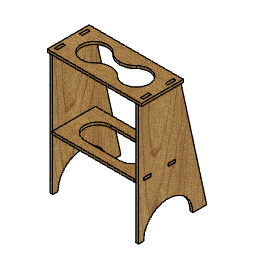
Prototipo_POMPE_2_0 (Autodesk Fusion 360 archive; units mm, degrees)
design "soporte_caños_corte_ v3"
Autodesk Fusion 360 part; units mm, degrees
sketch "Boceto1" plane through (0, 0, 0) normal (0, 0, 1) x (1, 0, 0)
  line L0 (0, 80) -> (0, -80) construction
  line L1 (180, 0) -> (180, -80)
  line L2 (180, 0) -> (180, 80)
  arc A0 (44.5386, -35.4614) -> (-44.5386, -35.4614) centre (0, -80) ccw
  arc A1 (-44.5386, 35.4614) -> (-44.5386, -35.4614) centre (-80, 0) ccw
  arc A2 (-44.5386, 35.4614) -> (44.5386, 35.4614) centre (0, 80) ccw
  arc A3 (44.5386, -35.4614) -> (44.5386, 35.4614) centre (80, 0) ccw
  line L3 (0, 0) -> (84.5309, 0)
  line L4 (-158.4928, 60.1913) -> (-158.4928, 34.434)
  line L5 (-180, 0) -> (-180, -80)
  line L6 (-166.3715, 62.3127) -> (-160.6141, 62.3127)
  line L7 (-180, 0) -> (-180, 80)
  line L8 (-168.4928, 34.434) -> (-168.4928, 60.1913)
  line L9 (-160.6141, 32.3127) -> (-166.3715, 32.3127)
  line L10 (-180, 80) -> (180, 80)
  line L11 (-180, -80) -> (180, -80)
  line L12 (-163.4928, 62.3127) -> (-163.4928, 32.3127)
  line L13 (-166.3715, 62.3127) -> (-160.1055, 62.3127) construction
  arc A4 (-166.3715, 62.3127) -> (-168.4928, 60.1913) centre (-167.4321, 61.252) ccw
  arc A5 (-158.4928, 60.1913) -> (-160.6141, 62.3127) centre (-159.5534, 61.252) ccw
  line L14 (-163.4928, 47.3127) -> (-158.4928, 47.3127)
  arc A6 (-160.6141, 32.3127) -> (-158.4928, 34.434) centre (-159.5534, 33.3733) ccw
  arc A7 (-168.4928, 34.434) -> (-166.3715, 32.3127) centre (-167.4321, 33.3733) ccw
  arc A8 (158.4928, 34.434) -> (160.6141, 32.3127) centre (159.5534, 33.3733) ccw
  line L15 (160.6141, 32.3127) -> (166.3715, 32.3127)
  arc A9 (166.3715, 32.3127) -> (168.4928, 34.434) centre (167.4321, 33.3733) ccw
  line L16 (168.4928, 34.434) -> (168.4928, 60.1913)
  arc A10 (168.4928, 60.1913) -> (166.3715, 62.3127) centre (167.4321, 61.252) ccw
  line L17 (166.3715, 62.3127) -> (160.6141, 62.3127)
  arc A11 (160.6141, 62.3127) -> (158.4928, 60.1913) centre (159.5534, 61.252) ccw
  line L18 (158.4928, 60.1913) -> (158.4928, 34.434)
  line L19 (166.3715, -62.3127) -> (160.6141, -62.3127)
  arc A12 (158.4928, -60.1913) -> (160.6141, -62.3127) centre (159.5534, -61.252) ccw
  line L20 (158.4928, -60.1913) -> (158.4928, -34.434)
  arc A13 (160.6141, -32.3127) -> (158.4928, -34.434) centre (159.5534, -33.3733) ccw
  line L21 (160.6141, -32.3127) -> (166.3715, -32.3127)
  arc A14 (168.4928, -34.434) -> (166.3715, -32.3127) centre (167.4321, -33.3733) ccw
  line L22 (168.4928, -34.434) -> (168.4928, -60.1913)
  arc A15 (166.3715, -62.3127) -> (168.4928, -60.1913) centre (167.4321, -61.252) ccw
  arc A16 (-158.4928, -34.434) -> (-160.6141, -32.3127) centre (-159.5534, -33.3733) ccw
  line L23 (-160.6141, -32.3127) -> (-166.3715, -32.3127)
  arc A17 (-166.3715, -32.3127) -> (-168.4928, -34.434) centre (-167.4321, -33.3733) ccw
  line L24 (-168.4928, -34.434) -> (-168.4928, -60.1913)
  arc A18 (-168.4928, -60.1913) -> (-166.3715, -62.3127) centre (-167.4321, -61.252) ccw
  line L25 (-166.3715, -62.3127) -> (-160.6141, -62.3127)
  arc A19 (-160.6141, -62.3127) -> (-158.4928, -60.1913) centre (-159.5534, -61.252) ccw
  line L26 (-158.4928, -60.1913) -> (-158.4928, -34.434)
  point P0 (-180.15, 0)
  dimension "d29" = 3
  dimension "d37" = 10
  constraint vertical L0
  constraint coincident L3.start origin
  constraint perpendicular L0 L3
  constraint symmetric L0 L1.start L5.start
  constraint symmetric L0 L1.end L5.end
  constraint symmetric L0 L2.end L7.end
  constraint perpendicular L2 L10
  constraint perpendicular L1 L11
  constraint perpendicular L9 L12
  constraint horizontal L13
  constraint symmetric L12 L8.end L4.start
  constraint symmetric L12 L6.start L6.end
  constraint symmetric L12 A4 A5
  constraint midpoint L12 L14.start
  constraint perpendicular L12 L14
  constraint symmetric L8.end L14 L8.start
  constraint symmetric L6.start L14 L9.end
  constraint symmetric A4 L14 A7
  constraint symmetric L6.end L14 L9.start
  constraint symmetric L4.start L14 L4.end
  constraint symmetric A5 L14 A6
  constraint coincident L6 L12.start
  constraint coincident L9 L12.end
  constraint symmetric L0 L8.end L16.end
  constraint symmetric L0 L6.start A10.end
  constraint symmetric L0 A4 A10
  constraint symmetric L0 L6.end L17.end
  constraint symmetric L0 L4.start A11.end
  constraint symmetric L0 A5 A11
  constraint symmetric L0 L4.end A8.start
  constraint symmetric L0 L9.start A8.end
  constraint symmetric L0 A6 A8
  constraint symmetric L0 L9.end L15.end
  constraint symmetric L0 L8.start A9.end
  constraint symmetric L0 A7 A9
  constraint symmetric L3 L8.end L24.end
  constraint symmetric L3 L6.start A18.end
  constraint symmetric L3 A4 A18
  constraint symmetric L3 L6.end L25.end
  constraint symmetric L3 L4.start A19.end
  constraint symmetric L3 A5 A19
  constraint symmetric L3 L4.end A16.start
  constraint symmetric L3 L9.start A16.end
  constraint symmetric L3 A6 A16
  constraint symmetric L3 L9.end L23.end
  constraint symmetric L3 L8.start A17.end
  constraint symmetric L3 A7 A17
  constraint symmetric L3 A8.end A13.start
  constraint symmetric L3 A8.start L20.end
  constraint symmetric L3 A8 A13
  constraint symmetric L3 L15.end L21.end
  constraint symmetric L3 A9.end A14.start
  constraint symmetric L3 A9 A14
  constraint symmetric L3 L16.end L22.end
  constraint symmetric L3 A10.end L19.start
  constraint symmetric L3 A10 A15
  constraint symmetric L3 L17.end L19.end
  constraint symmetric L3 A11.end A12.start
  constraint symmetric L3 A11 A12
  constraint coincident L0.end A0.centre
  constraint coincident L0.start A2.centre
  constraint horizontal L14
  constraint midpoint L4 L14.end
  measures "d29" diameter of A4
  measures "d37" distance of L4 L8
sketch "Boceto2" plane through (0, 0, 0) normal (0, 0, 1) x (1, 0, 0)
  line L0 (-158.6799, -83.0083) -> (0, -83.0083)
  arc A0 (-66.8983, 50.15) -> (-66.8983, -50.15) centre (-66.8983, 0) ccw
  line L1 (-66.8983, 50.15) -> (0, 50.15)
  line L2 (-66.8983, -50.15) -> (0, -50.15)
  line L3 (-158.6799, -62.4727) -> (-158.6799, -83.0083)
  line L4 (-169.0788, -33.0938) -> (-169.0788, -60.3514)
  line L5 (-160.8013, -33.0938) -> (-169.0788, -33.0938)
  line L6 (-169.0788, -60.3514) -> (-160.8013, -60.3514)
  line L7 (0, 0) -> (-158.6799, 0)
  line L8 (0, 0) -> (0, -83.0083)
  line L9 (-158.6799, -30.9725) -> (-158.6799, 0)
  arc A1 (-160.8013, -33.0938) -> (-158.6799, -30.9725) centre (-159.7406, -32.0332) ccw
  line L10 (-158.6799, -33.0938) -> (-159.7406, -32.0332) construction
  line L11 (-169.0788, -46.7226) -> (-158.6799, -46.7226)
  arc A2 (-158.6799, -62.4727) -> (-160.8013, -60.3514) centre (-159.7406, -61.412) ccw
  line L12 (-158.6799, 83.0083) -> (0, 83.0083)
  line L13 (-158.6799, 62.4727) -> (-158.6799, 83.0083)
  arc A3 (-160.8013, 60.3514) -> (-158.6799, 62.4727) centre (-159.7406, 61.412) ccw
  line L14 (-169.0788, 60.3514) -> (-160.8013, 60.3514)
  line L15 (-169.0788, 33.0938) -> (-169.0788, 60.3514)
  line L16 (-160.8013, 33.0938) -> (-169.0788, 33.0938)
  arc A4 (-158.6799, 30.9725) -> (-160.8013, 33.0938) centre (-159.7406, 32.0332) ccw
  line L17 (-158.6799, 30.9725) -> (-158.6799, 0)
  line L18 (158.6799, 83.0083) -> (0, 83.0083)
  line L19 (158.6799, 62.4727) -> (158.6799, 83.0083)
  arc A5 (158.6799, 62.4727) -> (160.8013, 60.3514) centre (159.7406, 61.412) ccw
  line L20 (169.0788, 60.3514) -> (160.8013, 60.3514)
  line L21 (169.0788, 33.0938) -> (169.0788, 60.3514)
  line L22 (160.8013, 33.0938) -> (169.0788, 33.0938)
  arc A6 (160.8013, 33.0938) -> (158.6799, 30.9725) centre (159.7406, 32.0332) ccw
  line L23 (158.6799, 30.9725) -> (158.6799, 0)
  line L24 (158.6799, -30.9725) -> (158.6799, 0)
  arc A7 (158.6799, -30.9725) -> (160.8013, -33.0938) centre (159.7406, -32.0332) ccw
  line L25 (160.8013, -33.0938) -> (169.0788, -33.0938)
  line L26 (169.0788, -33.0938) -> (169.0788, -60.3514)
  line L27 (169.0788, -60.3514) -> (160.8013, -60.3514)
  arc A8 (160.8013, -60.3514) -> (158.6799, -62.4727) centre (159.7406, -61.412) ccw
  line L28 (158.6799, -62.4727) -> (158.6799, -83.0083)
  line L29 (158.6799, -83.0083) -> (0, -83.0083)
  line L30 (66.8983, -50.15) -> (0, -50.15)
  arc A9 (66.8983, -50.15) -> (66.8983, 50.15) centre (66.8983, 0) ccw
  line L31 (66.8983, 50.15) -> (0, 50.15)
  dimension "d32" = 3
  constraint coincident A0 L1.start
  constraint coincident L1 A0.start
  constraint coincident L2 A0.end
  constraint coincident L7.start L8.start
  constraint horizontal L7
  constraint coincident A0.end L2.start
  constraint coincident A0.centre L7
  constraint horizontal L1
  constraint horizontal L2
  constraint tangent A0 L1
  constraint tangent A0 L2
  constraint horizontal L0
  constraint collinear L3 L9
  constraint vertical L3
  constraint coincident L10.start A1
  constraint horizontal L5
  constraint horizontal L6
  constraint vertical L4
  constraint vertical L8
  constraint coincident L2.end L8
  constraint coincident A1.centre L10.end
  constraint symmetric L5.start L9.start L10
  constraint midpoint L4 L11.start
  constraint perpendicular L4 L11
  constraint symmetric L5.start L11 L6.end
  constraint symmetric L9.start L11 L3.start
  constraint symmetric A1 L11 A2
  constraint symmetric L0.end L7 L12.end
  constraint symmetric L4.end L7 L14.start
  constraint symmetric L0.start L7 L12.start
  constraint symmetric L4.start L7 L15.start
  constraint symmetric L9.end L7 L17.end
  constraint symmetric L7 L5.start L16.start
  constraint symmetric L7 L9.start A4.start
  constraint symmetric L7 A1 A4
  constraint symmetric L7 L6.end A3.start
  constraint symmetric L7 L3.start L13.start
  constraint symmetric L7 A2 A3
  constraint symmetric A0 L8 A9
  constraint symmetric A0.start L8 A9.end
  constraint symmetric L1.end L8 L31.end
  constraint symmetric A0.end L8 L30.start
  constraint symmetric L2.end L8 L30.end
  constraint symmetric L0.end L8 L29.end
  constraint symmetric L4.end L8 L26.end
  constraint symmetric L0.start L8 L28.end
  constraint symmetric L4.start L8 L25.end
  constraint symmetric L7.end L8 L23.end
  constraint symmetric L8 L5.start A7.end
  constraint symmetric L8 L9.start L24.start
  constraint symmetric L8 A1 A7
  constraint symmetric L8 L6.end L27.end
  constraint symmetric L8 L3.start A8.end
  constraint symmetric L8 A2 A8
  constraint symmetric L8 L12.start L18.start
  constraint symmetric L8 L12.end L18.end
  constraint symmetric L8 L13.start L19.start
  constraint symmetric L8 A3.start A5.end
  constraint symmetric L8 A3 A5
  constraint symmetric L8 L14.start L20.start
  constraint symmetric L8 L15.start L21.start
  constraint symmetric L8 L16.start L22.start
  constraint symmetric L8 A4.start A6.end
  constraint symmetric L8 A4 A6
  constraint symmetric L8 L7.end L23.end
  measures "d32" distance of L5.start L9.start
extrude "Extruir1" add sketch "Boceto1" along normal blind 10 makes body 1
move_body "Desplazar1" bodies 1 to x (1, 0, 0) y (0, 1, 0) z (0, 0, 1) at (0, 0, 460)
extrude "Extruir2" add sketch "Boceto2" along normal blind 10 separate body contours L0 A0 L2 L3 L4 L5 L6 L7 L8 L9 A1 A2 | A0 L1 L7 L8 L12 L13 A3 L14 L15 L16 A4 L17 L18 L19 A5 L20 L21 L22 A6 L23 L24 A7 L25 L26 L27 A8 L28 L29 L30 A9 L31 makes body 2
move_body "Desplazar2" bodies 2 to x (1, 0, 0) y (0, 1, 0) z (0, 0, 1) at (0, 0, 200)
ref_plane "PlanoDeObra1" through (-158.6799, 0, 0) normal (1, 0, 0) x (0, 1, 0)
sketch "Boceto3" plane through (-158.6799, 0, 0) normal (1, 0, 0) x (0, 1, 0)
  line L0 (-80, 460) -> (-80, 0)
  line L1 (80, 460) -> (180, 0)
  line L2 (-80, 0) -> (-60.2742, 0)
  line L3 (127.088, 0) -> (180, 0)
  arc A0 (127.088, 0) -> (-60.2742, 0) centre (33.4069, 0) ccw
  line L4 (80, 460) -> (-80, 460)
  line L5 (60.3514, 200) -> (33.0938, 200)
  line L6 (33.0938, 200) -> (33.0938, 210)
  line L7 (33.0938, 210) -> (60.3514, 210)
  line L8 (60.3514, 210) -> (60.3514, 200)
  line L9 (-33.0938, 200) -> (-60.3514, 200)
  line L10 (-60.3514, 200) -> (-60.3514, 210)
  line L11 (-60.3514, 210) -> (-33.0938, 210)
  line L12 (-33.0938, 210) -> (-33.0938, 200)
  line L13 (62.3127, 470) -> (62.3127, 462.1213)
  line L14 (32.3127, 470) -> (32.3127, 462.1213)
  line L15 (-32.3127, 470) -> (-32.3127, 462.1213)
  line L16 (-62.3127, 470) -> (-62.3127, 462.1213)
  arc A1 (62.3127, 462.1213) -> (64.434, 460) centre (63.3733, 461.0607) ccw
  line L17 (62.3127, 460) -> (63.3733, 461.0607) construction
  line L18 (62.3127, 470) -> (32.3127, 470)
  line L19 (-32.3127, 470) -> (-62.3127, 470)
  line L20 (47.3127, 470) -> (47.3127, 460)
  arc A2 (30.1913, 460) -> (32.3127, 462.1213) centre (31.252, 461.0607) ccw
  line L21 (0, 460) -> (0, 470.5276)
  arc A3 (-64.434, 460) -> (-62.3127, 462.1213) centre (-63.3733, 461.0607) ccw
  arc A4 (-32.3127, 462.1213) -> (-30.1913, 460) centre (-31.252, 461.0607) ccw
  arc A5 (60.3514, 207.8787) -> (58.2301, 210) centre (59.2907, 208.9393) ccw
  line L22 (60.3514, 210) -> (59.2907, 208.9393)
  line L23 (46.7226, 210) -> (46.7226, 200)
  arc A6 (35.2152, 210) -> (33.0938, 207.8787) centre (34.1545, 208.9393) ccw
  line L24 (60.3514, 205) -> (33.0938, 205)
  arc A7 (58.2301, 200) -> (60.3514, 202.1213) centre (59.2907, 201.0607) ccw
  arc A8 (33.0938, 202.1213) -> (35.2152, 200) centre (34.1545, 201.0607) ccw
  arc A9 (-60.3514, 202.1213) -> (-58.2301, 200) centre (-59.2907, 201.0607) ccw
  arc A10 (-58.2301, 210) -> (-60.3514, 207.8787) centre (-59.2907, 208.9393) ccw
  arc A11 (-33.0938, 207.8787) -> (-35.2152, 210) centre (-34.1545, 208.9393) ccw
  arc A12 (-35.2152, 200) -> (-33.0938, 202.1213) centre (-34.1545, 201.0607) ccw
  point P0 (32.3127, 460)
  point P1 (32.3127, 470)
  point P2 (62.3127, 460)
  point P3 (62.3127, 470)
  point P4 (-62.3127, 470)
  point P5 (-32.3127, 470)
  point P6 (-62.3127, 460)
  point P7 (-32.3127, 460)
  dimension "d20" = 460
  dimension "d21" = 260
  dimension "d33" = 45
  dimension "d34" = 3
  dimension "d35" = 45
  dimension "d36" = 3
  constraint perpendicular L0 L2
  constraint coincident A0.centre L2
  constraint collinear L2 L3
  constraint coincident L1.start L4.start
  constraint coincident L0.start L4.end
  constraint coincident P3 L13.start
  constraint coincident P2 L17.start
  constraint coincident P1 L14.start
  constraint coincident P5 L15.start
  constraint coincident P4 L16.start
  constraint coincident P2 A1
  constraint coincident L4 A1.end
  constraint coincident A1.centre L17.end
  constraint midpoint L18 L20.start
  constraint coincident L4 L20.end
  constraint perpendicular L4 L20
  constraint symmetric L13.end L20 L14.end
  constraint symmetric A1.end L20 A2.start
  constraint symmetric A1 L20 A2
  constraint midpoint L4 L21.start
  constraint perpendicular L4 L21
  constraint symmetric L13.end L21 L16.end
  constraint symmetric A1.end L21 A3.start
  constraint symmetric A1 L21 A3
  constraint symmetric L14.end L21 L15.end
  constraint symmetric A2.start L21 A4.end
  constraint symmetric A2 L21 A4
  constraint vertical L13
  constraint coincident L7.end A5
  constraint coincident L7 A5.end
  constraint coincident L8 A5.start
  constraint coincident L7.end L8.start
  constraint coincident A5.centre L22.end
  constraint midpoint L7 L23.start
  constraint coincident L5 L23.end
  constraint vertical L23
  constraint symmetric A5.start L23 A6.end
  constraint symmetric A5.end L23 A6.start
  constraint symmetric A5 L23 A6
  constraint midpoint L8 L24.start
  constraint midpoint L6 L24.end
  constraint symmetric A5.start L24 A7.end
  constraint symmetric A5.end L24 A7.start
  constraint symmetric A5 L24 A7
  constraint symmetric A6.end L24 A8.start
  constraint symmetric A6.start L24 A8.end
  constraint symmetric A6 L24 A8
  constraint symmetric L21 A5.start A10.end
  constraint symmetric L21 A5.end A10.start
  constraint symmetric L21 A5 A10
  constraint symmetric L21 A6.end A11.start
  constraint symmetric L21 A6.start A11.end
  constraint symmetric L21 A6 A11
  constraint symmetric L21 A7.end A9.start
  constraint symmetric L21 A7.start A9.end
  constraint symmetric L21 A7 A9
  constraint symmetric L21 A8.end A12.start
  constraint symmetric L21 A8.start A12.end
  constraint symmetric L21 A8 A12
  measures "d20" distance of L0.end L0.start
  measures "d21" distance of L0.end L1.end
  measures "d33" angle of L4 L17
  measures "d34" distance of L13.end A1.end
  measures "d35" angle of L7 L22
  measures "d36" distance of A5.start A5.end
extrude "Extruir3" add sketch "Boceto3" against normal blind 10 separate body contours L0 L1 L2 L3 A0 L4 A1 A2 A3 A4 | L4 L15 L16 L19 A3 A4 | L4 L13 A1 L18 L20 | L4 L14 L18 L20 A2 makes body 3
mirror "Simetría1" about plane through (0, 0, 0) normal (1, 0, 0) of bodies 3 makes body 4
equation "diametro_caño = 100 mm"
equation "holgura = 0,15 mm"
equation "espezor_madera = 10 mm"
equation "d15 = espezor_madera"
equation "d17 = espezor_madera"
equation "d22 = -espezor_madera"
equation "d37 = espezor_madera"
